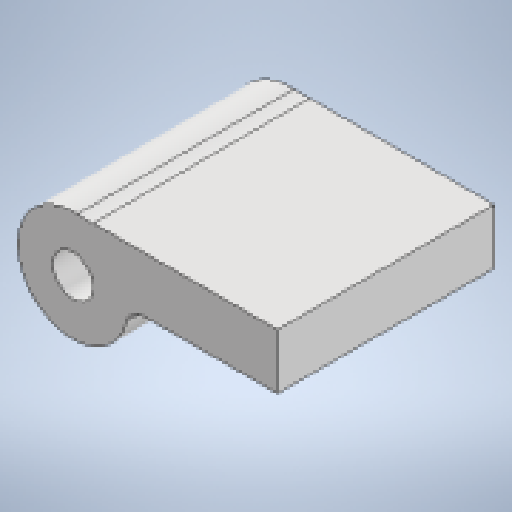
# Autodesk Inventor part: innerhinge
Saved by Autodesk Inventor 2026 (Build 300175050, 175E)
## iProperties
Created: 2025-10-10
Part Number: innerhinge
Material: Generic
Document SubType Name: Modeling
Designer: Nicholas M
Density: 1 g/cm^3
Appearance: Default
Author: Nicholas M
Autodesk Inventor part; units mm, degrees
ref_plane "YZ Plane" through (0, 0, 0) normal (1, 0, 0) x (0, 1, 0)
ref_plane "XZ Plane" through (0, 0, 0) normal (0, 1, 0) x (-1, 0, 0)
ref_plane "XY Plane" through (0, 0, 0) normal (0, 0, 1) x (1, 0, 0)
sketch "Sketch1" plane through (0, 0, 0) normal (0, 0, 1) x (1, 0, 0)
  circle A0 centre (0, 0) radius 0.6985
  circle A1 centre (0, 0) radius 1.905
  line L0 (0.6985, 0) -> (7.0485, 0)
  line L1 (7.0485, 0) -> (7.0485, 1.905)
  line L2 (7.0485, 1.905) -> (0.6985, 1.905)
  line L3 (0.6985, 1.905) -> (0.6985, 0)
  point P0 (0.6985, 1.7723)
  point P1 (1.905, 0)
  dimension "d0" = 1.397
  dimension "d1" = 3.81
  dimension "d4" = 6.35
  dimension "d5" = 1.905
  constraints: 8 end point, 2 coincident, 2 parallel, 1 centre point, 1 horizontal, 1 horizontal alignment, 1 perpendicular, 1 tangent, 2 other
  measures "d1" diameter of A1
  measures "d4" distance of L2.end L1.end
  measures "d5" distance of L1.end L0.end
extrude "Extrusion1" add sketch "Sketch1" along normal blind 7.62
fillet "Fillet1" radius 3.175 1 edges at (0.6985, 1.7723, 3.81)
fillet "Fillet2" radius 0.5292 1 edges at (1.905, 0, 3.81)
body "Solid1"
